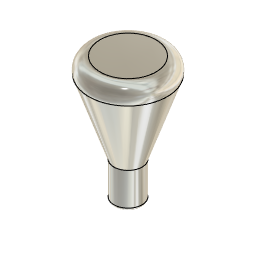
punchSetPin v1 (Autodesk Fusion 360 design; units mm, degrees)
Autodesk Fusion 360 part; units mm, degrees
sketch "Sketch1" plane through (0, 0, 0) normal (0, 0, 1) x (1, 0, 0)
  circle A0 centre (0, 0) radius 2.375
  dimension "d1" = 4.75
  constraint coincident A0.centre origin
  measures "d1" diameter of A0
extrude "Extrude1" add sketch "Sketch1" along normal blind 6
sketch "Sketch2" plane through (0, 0, 6) normal (0, 0, 1) x (-1, 0, 0)
  circle A0 centre (0, 0) radius 2.375
  line L0 (0, 0, 0) -> (0, 0, 15)
  circle A1 through (7.5, 0, 15) (-3.75, 6.4952, 15) (-3.75, -6.4952, 15)
  constraint coincident A0.centre origin
  measures "d4" distance of A0.centre origin
loft "Loft1" add profiles "Sketch2", "Sketch2" section 1 contours A1 in plane through (0, 0, 21) normal (0, 0, 1) section 2
fillet "Fillet1" radius 2 1 edges at (6.9925, -2.7121, 21)
fillet "Fillet2" radius 0.5 1 edges at (-2.2143, -0.8588, 0)
